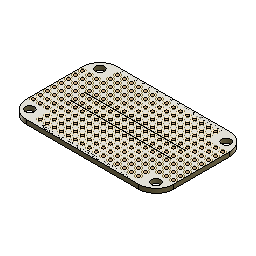
1214 Perma-Proto Small Mint (Autodesk Fusion 360 design; units mm, degrees)
Autodesk Fusion 360 part; units mm, degrees
sketch "sketch 305" plane through (0, 0, 0) normal (0, 0, 1) x (1, 0, 0)
  line L0 (-20.32, 16.51) -> (20.32, 16.51)
  arc A0 (26.67, 10.16) -> (20.32, 16.51) centre (20.32, 10.16) ccw
  line L1 (26.67, 10.16) -> (26.67, -10.16)
  arc A1 (20.32, -16.51) -> (26.67, -10.16) centre (20.32, -10.16) ccw
  line L2 (20.32, -16.51) -> (-20.32, -16.51)
  arc A2 (-26.67, -10.16) -> (-20.32, -16.51) centre (-20.32, -10.16) ccw
  line L3 (-26.67, -10.16) -> (-26.67, 10.16)
  arc A3 (-20.32, 16.51) -> (-26.67, 10.16) centre (-20.32, 10.16) ccw
  circle A4 centre (-22.86, 12.7) radius 1.6
  circle A5 centre (22.86, 12.7) radius 1.6
  circle A6 centre (-22.86, -12.7) radius 1.6
  circle A7 centre (22.86, -12.7) radius 1.6
extrude "Board" add sketch "sketch 305" along normal blind 1.57 makes body 1 in component "Board"
sketch "sketch 1943" plane through (0, 0, 0) normal (0, 0, 1) x (1, 0, 0)
  line L0 (-16.51, -26.67) -> (16.51, -26.67)
  line L1 (16.51, -26.67) -> (16.51, 26.67)
  line L2 (16.51, 26.67) -> (-16.51, 26.67)
  line L3 (-16.51, 26.67) -> (-16.51, -26.67)
extrude "ALTOIDSSMALLS" add sketch "sketch 1943" along normal blind 0.1 separate body makes body 2 in component "ALTOIDSSMALLS"
sketch "sketch 460" plane through (0, 0, 0) normal (0, 0, 1) x (1, 0, 0)
  circle A0 centre (-17.78, -13.97) radius 0.6
  circle A1 centre (-17.78, -11.43) radius 0.6
  circle A2 centre (-17.78, -8.89) radius 0.6
  circle A3 centre (-17.78, -6.35) radius 0.6
  circle A4 centre (-17.78, -3.81) radius 0.6
  circle A5 centre (-15.24, -13.97) radius 0.6
  circle A6 centre (-15.24, -11.43) radius 0.6
  circle A7 centre (-15.24, -8.89) radius 0.6
  circle A8 centre (-15.24, -6.35) radius 0.6
  circle A9 centre (-15.24, -3.81) radius 0.6
  circle A10 centre (-12.7, -13.97) radius 0.6
  circle A11 centre (-12.7, -11.43) radius 0.6
  circle A12 centre (-12.7, -8.89) radius 0.6
  circle A13 centre (-12.7, -6.35) radius 0.6
  circle A14 centre (-12.7, -3.81) radius 0.6
  circle A15 centre (-10.16, -13.97) radius 0.6
  circle A16 centre (-10.16, -11.43) radius 0.6
  circle A17 centre (-10.16, -8.89) radius 0.6
  circle A18 centre (-10.16, -6.35) radius 0.6
  circle A19 centre (-10.16, -3.81) radius 0.6
  circle A20 centre (-7.62, -13.97) radius 0.6
  circle A21 centre (-7.62, -11.43) radius 0.6
  circle A22 centre (-7.62, -8.89) radius 0.6
  circle A23 centre (-7.62, -6.35) radius 0.6
  circle A24 centre (-7.62, -3.81) radius 0.6
  circle A25 centre (-5.08, -13.97) radius 0.6
  circle A26 centre (-5.08, -11.43) radius 0.6
  circle A27 centre (-5.08, -8.89) radius 0.6
  circle A28 centre (-5.08, -6.35) radius 0.6
  circle A29 centre (-5.08, -3.81) radius 0.6
  circle A30 centre (0, -13.97) radius 0.6
  circle A31 centre (0, -11.43) radius 0.6
  circle A32 centre (0, -8.89) radius 0.6
  circle A33 centre (0, -6.35) radius 0.6
  circle A34 centre (0, -3.81) radius 0.6
  circle A35 centre (-2.54, -13.97) radius 0.6
  circle A36 centre (-2.54, -11.43) radius 0.6
  circle A37 centre (-2.54, -8.89) radius 0.6
  circle A38 centre (-2.54, -6.35) radius 0.6
  circle A39 centre (-2.54, -3.81) radius 0.6
  circle A40 centre (2.54, -13.97) radius 0.6
  circle A41 centre (2.54, -11.43) radius 0.6
  circle A42 centre (2.54, -8.89) radius 0.6
  circle A43 centre (2.54, -6.35) radius 0.6
  circle A44 centre (2.54, -3.81) radius 0.6
  circle A45 centre (5.08, -13.97) radius 0.6
  circle A46 centre (5.08, -11.43) radius 0.6
  circle A47 centre (5.08, -8.89) radius 0.6
  circle A48 centre (5.08, -6.35) radius 0.6
  circle A49 centre (5.08, -3.81) radius 0.6
  circle A50 centre (7.62, -13.97) radius 0.6
  circle A51 centre (7.62, -11.43) radius 0.6
  circle A52 centre (7.62, -8.89) radius 0.6
  circle A53 centre (7.62, -6.35) radius 0.6
  circle A54 centre (7.62, -3.81) radius 0.6
  circle A55 centre (10.16, -13.97) radius 0.6
  circle A56 centre (10.16, -11.43) radius 0.6
  circle A57 centre (10.16, -8.89) radius 0.6
  circle A58 centre (10.16, -6.35) radius 0.6
  circle A59 centre (10.16, -3.81) radius 0.6
  circle A60 centre (12.7, -13.97) radius 0.6
  circle A61 centre (12.7, -11.43) radius 0.6
  circle A62 centre (12.7, -8.89) radius 0.6
  circle A63 centre (12.7, -6.35) radius 0.6
  circle A64 centre (12.7, -3.81) radius 0.6
  circle A65 centre (15.24, -13.97) radius 0.6
  circle A66 centre (15.24, -11.43) radius 0.6
  circle A67 centre (15.24, -8.89) radius 0.6
  circle A68 centre (15.24, -6.35) radius 0.6
  circle A69 centre (15.24, -3.81) radius 0.6
  circle A70 centre (17.78, -13.97) radius 0.6
  circle A71 centre (17.78, -11.43) radius 0.6
  circle A72 centre (17.78, -8.89) radius 0.6
  circle A73 centre (17.78, -6.35) radius 0.6
  circle A74 centre (17.78, -3.81) radius 0.6
  circle A75 centre (17.78, 13.97) radius 0.6
  circle A76 centre (17.78, 11.43) radius 0.6
  circle A77 centre (17.78, 8.89) radius 0.6
  circle A78 centre (17.78, 6.35) radius 0.6
  circle A79 centre (17.78, 3.81) radius 0.6
  circle A80 centre (12.7, 13.97) radius 0.6
  circle A81 centre (12.7, 11.43) radius 0.6
  circle A82 centre (12.7, 8.89) radius 0.6
  circle A83 centre (12.7, 6.35) radius 0.6
  circle A84 centre (12.7, 3.81) radius 0.6
  circle A85 centre (15.24, 13.97) radius 0.6
  circle A86 centre (15.24, 11.43) radius 0.6
  circle A87 centre (15.24, 8.89) radius 0.6
  circle A88 centre (15.24, 6.35) radius 0.6
  circle A89 centre (15.24, 3.81) radius 0.6
  circle A90 centre (10.16, 13.97) radius 0.6
  circle A91 centre (10.16, 11.43) radius 0.6
  circle A92 centre (10.16, 8.89) radius 0.6
  circle A93 centre (10.16, 6.35) radius 0.6
  circle A94 centre (10.16, 3.81) radius 0.6
  circle A95 centre (7.62, 13.97) radius 0.6
  circle A96 centre (7.62, 11.43) radius 0.6
  circle A97 centre (7.62, 8.89) radius 0.6
  circle A98 centre (7.62, 6.35) radius 0.6
  circle A99 centre (7.62, 3.81) radius 0.6
  circle A100 centre (2.54, 13.97) radius 0.6
  circle A101 centre (2.54, 11.43) radius 0.6
  circle A102 centre (2.54, 8.89) radius 0.6
  circle A103 centre (2.54, 6.35) radius 0.6
  circle A104 centre (2.54, 3.81) radius 0.6
  circle A105 centre (5.08, 13.97) radius 0.6
  circle A106 centre (5.08, 11.43) radius 0.6
  circle A107 centre (5.08, 8.89) radius 0.6
  circle A108 centre (5.08, 6.35) radius 0.6
  circle A109 centre (5.08, 3.81) radius 0.6
  circle A110 centre (0, 13.97) radius 0.6
  circle A111 centre (0, 11.43) radius 0.6
  circle A112 centre (0, 8.89) radius 0.6
  circle A113 centre (0, 3.81) radius 0.6
  circle A114 centre (0, 6.35) radius 0.6
  circle A115 centre (-2.54, 13.97) radius 0.6
  circle A116 centre (-2.54, 11.43) radius 0.6
  circle A117 centre (-2.54, 8.89) radius 0.6
  circle A118 centre (-2.54, 6.35) radius 0.6
  circle A119 centre (-2.54, 3.81) radius 0.6
  circle A120 centre (-5.08, 13.97) radius 0.6
  circle A121 centre (-5.08, 11.43) radius 0.6
  circle A122 centre (-5.08, 8.89) radius 0.6
  circle A123 centre (-5.08, 6.35) radius 0.6
  circle A124 centre (-5.08, 3.81) radius 0.6
  circle A125 centre (-7.62, 13.97) radius 0.6
  circle A126 centre (-7.62, 11.43) radius 0.6
  circle A127 centre (-7.62, 8.89) radius 0.6
  circle A128 centre (-7.62, 6.35) radius 0.6
  circle A129 centre (-7.62, 3.81) radius 0.6
  circle A130 centre (-12.7, 13.97) radius 0.6
  circle A131 centre (-12.7, 11.43) radius 0.6
  circle A132 centre (-12.7, 8.89) radius 0.6
  circle A133 centre (-12.7, 6.35) radius 0.6
  circle A134 centre (-12.7, 3.81) radius 0.6
  circle A135 centre (-10.16, 13.97) radius 0.6
  circle A136 centre (-10.16, 11.43) radius 0.6
  circle A137 centre (-10.16, 8.89) radius 0.6
  circle A138 centre (-10.16, 6.35) radius 0.6
  circle A139 centre (-10.16, 3.81) radius 0.6
  circle A140 centre (-15.24, 13.97) radius 0.6
  circle A141 centre (-15.24, 11.43) radius 0.6
  circle A142 centre (-15.24, 8.89) radius 0.6
  circle A143 centre (-15.24, 6.35) radius 0.6
  circle A144 centre (-15.24, 3.81) radius 0.6
  circle A145 centre (-17.78, 13.97) radius 0.6
  circle A146 centre (-17.78, 11.43) radius 0.6
  circle A147 centre (-17.78, 8.89) radius 0.6
  circle A148 centre (-17.78, 6.35) radius 0.6
  circle A149 centre (-17.78, 3.81) radius 0.6
  circle A150 centre (17.78, -1.27) radius 0.6
  circle A151 centre (15.24, -1.27) radius 0.6
  circle A152 centre (12.7, -1.27) radius 0.6
  circle A153 centre (10.16, -1.27) radius 0.6
  circle A154 centre (7.62, -1.27) radius 0.6
  circle A155 centre (5.08, -1.27) radius 0.6
  circle A156 centre (0, -1.27) radius 0.6
  circle A157 centre (2.54, -1.27) radius 0.6
  circle A158 centre (-2.54, -1.27) radius 0.6
  circle A159 centre (-5.08, -1.27) radius 0.6
  circle A160 centre (-7.62, -1.27) radius 0.6
  circle A161 centre (-10.16, -1.27) radius 0.6
  circle A162 centre (-12.7, -1.27) radius 0.6
  circle A163 centre (-15.24, -1.27) radius 0.6
  circle A164 centre (-17.78, -1.27) radius 0.6
  circle A165 centre (17.78, 1.27) radius 0.6
  circle A166 centre (15.24, 1.27) radius 0.6
  circle A167 centre (12.7, 1.27) radius 0.6
  circle A168 centre (10.16, 1.27) radius 0.6
  circle A169 centre (7.62, 1.27) radius 0.6
  circle A170 centre (5.08, 1.27) radius 0.6
  circle A171 centre (0, 1.27) radius 0.6
  circle A172 centre (2.54, 1.27) radius 0.6
  circle A173 centre (-2.54, 1.27) radius 0.6
  circle A174 centre (-5.08, 1.27) radius 0.6
  circle A175 centre (-7.62, 1.27) radius 0.6
  circle A176 centre (-10.16, 1.27) radius 0.6
  circle A177 centre (-12.7, 1.27) radius 0.6
  circle A178 centre (-15.24, 1.27) radius 0.6
  circle A179 centre (-17.78, 1.27) radius 0.6
  circle A180 centre (-20.32, 8.89) radius 0.6
  circle A181 centre (-20.32, 6.35) radius 0.6
  circle A182 centre (-20.32, 3.81) radius 0.6
  circle A183 centre (-22.86, 3.81) radius 0.6
  circle A184 centre (-22.86, 6.35) radius 0.6
  circle A185 centre (-22.86, 8.89) radius 0.6
  circle A186 centre (-25.4, 8.89) radius 0.6
  circle A187 centre (-25.4, 6.35) radius 0.6
  circle A188 centre (-25.4, 3.81) radius 0.6
  circle A189 centre (-25.4, 1.27) radius 0.6
  circle A190 centre (-22.86, 1.27) radius 0.6
  circle A191 centre (-20.32, 1.27) radius 0.6
  circle A192 centre (-20.32, -1.27) radius 0.6
  circle A193 centre (-22.86, -1.27) radius 0.6
  circle A194 centre (-25.4, -1.27) radius 0.6
  circle A195 centre (-25.4, -3.81) radius 0.6
  circle A196 centre (-22.86, -3.81) radius 0.6
  circle A197 centre (-20.32, -3.81) radius 0.6
  circle A198 centre (-20.32, -6.35) radius 0.6
  circle A199 centre (-22.86, -6.35) radius 0.6
  circle A200 centre (-25.4, -6.35) radius 0.6
  circle A201 centre (-25.4, -8.89) radius 0.6
  circle A202 centre (-22.86, -8.89) radius 0.6
  circle A203 centre (-20.32, -8.89) radius 0.6
  circle A204 centre (20.32, 8.89) radius 0.6
  circle A205 centre (20.32, 6.35) radius 0.6
  circle A206 centre (20.32, 3.81) radius 0.6
  circle A207 centre (22.86, 3.81) radius 0.6
  circle A208 centre (22.86, 6.35) radius 0.6
  circle A209 centre (22.86, 8.89) radius 0.6
  circle A210 centre (25.4, 8.89) radius 0.6
  circle A211 centre (25.4, 6.35) radius 0.6
  circle A212 centre (25.4, 3.81) radius 0.6
  circle A213 centre (25.4, 1.27) radius 0.6
  circle A214 centre (25.4, -1.27) radius 0.6
  circle A215 centre (25.4, -3.81) radius 0.6
  circle A216 centre (25.4, -6.35) radius 0.6
  circle A217 centre (25.4, -8.89) radius 0.6
  circle A218 centre (22.86, -8.89) radius 0.6
  circle A219 centre (20.32, -8.89) radius 0.6
  circle A220 centre (22.86, -6.35) radius 0.6
  circle A221 centre (20.32, -6.35) radius 0.6
  circle A222 centre (20.32, -3.81) radius 0.6
  circle A223 centre (22.86, -3.81) radius 0.6
  circle A224 centre (22.86, -1.27) radius 0.6
  circle A225 centre (20.32, -1.27) radius 0.6
  circle A226 centre (20.32, 1.27) radius 0.6
  circle A227 centre (22.86, 1.27) radius 0.6
extrude "Extrude2" cut sketch "sketch 460" along normal blind 1.57 bodies 1 in component "Board"
component "PCB Component" placed x (1, 0, 0) y (0, 1, 0) z (0, 0, 1) at (0, 0, 0)
component "Board" placed x (1, 0, 0) y (0, 1, 0) z (0, 0, 1) at (0, 0, 0) in component "PCB Component"
component "ALTOIDSSMALLS" placed x (0, 1, 0) y (-1, 0, 0) z (0, 0, 1) at (0, 0, 1.57) in component "PCB Component"
named bodies: "Board", "ALTOIDSSMALLS"
